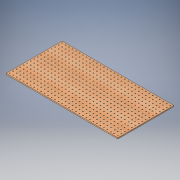
# Autodesk Inventor part: LedBoard
Saved by Autodesk Inventor 2016 (Build 200138000, 138)
## iProperties
Created: 2016-02-08
Part Number: LedBoard
Material: Wood (Birch)
Document SubType Name: Modeling
Designer: ron
Density: 0.55 g/cm^3
Appearance: Birch - Natural Polished
Mass: 4901.48 g
Surface Area: 16574.3 cm^2
Volume: 8911.78 cm^3
Author: ron
Autodesk Inventor part; units mm, degrees
ref_plane "YZ Plane" through (0, 0, 0) normal (1, 0, 0) x (0, 1, 0)
ref_plane "XZ Plane" through (0, 0, 0) normal (0, 1, 0) x (-1, 0, 0)
ref_plane "XY Plane" through (0, 0, 0) normal (0, 0, 1) x (1, 0, 0)
sketch "Sketch1" plane through (0, 0, 0) normal (0, 1, 0) x (-1, 0, 0)
  line L0 (0, 0) -> (1219.2, 0)
  line L1 (1219.2, 0) -> (1219.2, -609.6)
  line L2 (1219.2, -609.6) -> (0, -609.6)
  line L3 (0, -609.6) -> (0, 0)
  circle A0 centre (1200.15, -590.55) radius 5.08
  circle A1 centre (1200.15, -552.45) radius 5.08
  circle A2 centre (1200.15, -514.35) radius 5.08
  circle A3 centre (1200.15, -476.25) radius 5.08
  circle A4 centre (1200.15, -438.15) radius 5.08
  circle A5 centre (1200.15, -400.05) radius 5.08
  circle A6 centre (1200.15, -361.95) radius 5.08
  circle A7 centre (1200.15, -323.85) radius 5.08
  circle A8 centre (1200.15, -285.75) radius 5.08
  circle A9 centre (1200.15, -247.65) radius 5.08
  circle A10 centre (1200.15, -209.55) radius 5.08
  circle A11 centre (1200.15, -171.45) radius 5.08
  circle A12 centre (1200.15, -133.35) radius 5.08
  circle A13 centre (1200.15, -95.25) radius 5.08
  circle A14 centre (1200.15, -57.15) radius 5.08
  circle A15 centre (1200.15, -19.05) radius 5.08
  circle A16 centre (1162.05, -590.55) radius 5.08
  circle A17 centre (1162.05, -552.45) radius 5.08
  circle A18 centre (1162.05, -514.35) radius 5.08
  circle A19 centre (1162.05, -476.25) radius 5.08
  circle A20 centre (1162.05, -438.15) radius 5.08
  circle A21 centre (1162.05, -400.05) radius 5.08
  circle A22 centre (1162.05, -361.95) radius 5.08
  circle A23 centre (1162.05, -323.85) radius 5.08
  circle A24 centre (1162.05, -171.45) radius 5.08
  circle A25 centre (1162.05, -209.55) radius 5.08
  circle A26 centre (1162.05, -247.65) radius 5.08
  circle A27 centre (1162.05, -285.75) radius 5.08
  circle A28 centre (1162.05, -133.35) radius 5.08
  circle A29 centre (1162.05, -95.25) radius 5.08
  circle A30 centre (1162.05, -57.15) radius 5.08
  circle A31 centre (1162.05, -19.05) radius 5.08
  circle A32 centre (1123.95, -590.55) radius 5.08
  circle A33 centre (1123.95, -552.45) radius 5.08
  circle A34 centre (1123.95, -514.35) radius 5.08
  circle A35 centre (1123.95, -476.25) radius 5.08
  circle A36 centre (1123.95, -438.15) radius 5.08
  circle A37 centre (1123.95, -400.05) radius 5.08
  circle A38 centre (1123.95, -361.95) radius 5.08
  circle A39 centre (1123.95, -323.85) radius 5.08
  circle A40 centre (1123.95, -171.45) radius 5.08
  circle A41 centre (1123.95, -209.55) radius 5.08
  circle A42 centre (1123.95, -247.65) radius 5.08
  circle A43 centre (1123.95, -285.75) radius 5.08
  circle A44 centre (1123.95, -133.35) radius 5.08
  circle A45 centre (1123.95, -95.25) radius 5.08
  circle A46 centre (1123.95, -57.15) radius 5.08
  circle A47 centre (1123.95, -19.05) radius 5.08
  circle A48 centre (1085.85, -590.55) radius 5.08
  circle A49 centre (1085.85, -552.45) radius 5.08
  circle A50 centre (1085.85, -514.35) radius 5.08
  circle A51 centre (1085.85, -476.25) radius 5.08
  circle A52 centre (1085.85, -438.15) radius 5.08
  circle A53 centre (1085.85, -400.05) radius 5.08
  circle A54 centre (1085.85, -361.95) radius 5.08
  circle A55 centre (1085.85, -323.85) radius 5.08
  circle A56 centre (1085.85, -171.45) radius 5.08
  circle A57 centre (1085.85, -209.55) radius 5.08
  circle A58 centre (1085.85, -247.65) radius 5.08
  circle A59 centre (1085.85, -285.75) radius 5.08
  circle A60 centre (1085.85, -133.35) radius 5.08
  circle A61 centre (1085.85, -95.25) radius 5.08
  circle A62 centre (1085.85, -57.15) radius 5.08
  circle A63 centre (1085.85, -19.05) radius 5.08
  circle A64 centre (1047.75, -590.55) radius 5.08
  circle A65 centre (1047.75, -552.45) radius 5.08
  circle A66 centre (1047.75, -514.35) radius 5.08
  circle A67 centre (1047.75, -476.25) radius 5.08
  circle A68 centre (1047.75, -438.15) radius 5.08
  circle A69 centre (1047.75, -400.05) radius 5.08
  circle A70 centre (1047.75, -361.95) radius 5.08
  circle A71 centre (1047.75, -323.85) radius 5.08
  circle A72 centre (1047.75, -171.45) radius 5.08
  circle A73 centre (1047.75, -209.55) radius 5.08
  circle A74 centre (1047.75, -247.65) radius 5.08
  circle A75 centre (1047.75, -285.75) radius 5.08
  circle A76 centre (1047.75, -133.35) radius 5.08
  circle A77 centre (1047.75, -95.25) radius 5.08
  circle A78 centre (1047.75, -57.15) radius 5.08
  circle A79 centre (1047.75, -19.05) radius 5.08
  circle A80 centre (1009.65, -590.55) radius 5.08
  circle A81 centre (1009.65, -552.45) radius 5.08
  circle A82 centre (1009.65, -514.35) radius 5.08
  circle A83 centre (1009.65, -476.25) radius 5.08
  circle A84 centre (1009.65, -438.15) radius 5.08
  circle A85 centre (1009.65, -400.05) radius 5.08
  circle A86 centre (1009.65, -361.95) radius 5.08
  circle A87 centre (1009.65, -323.85) radius 5.08
  circle A88 centre (1009.65, -171.45) radius 5.08
  circle A89 centre (1009.65, -209.55) radius 5.08
  circle A90 centre (1009.65, -247.65) radius 5.08
  circle A91 centre (1009.65, -285.75) radius 5.08
  circle A92 centre (1009.65, -133.35) radius 5.08
  circle A93 centre (1009.65, -95.25) radius 5.08
  circle A94 centre (1009.65, -57.15) radius 5.08
  circle A95 centre (1009.65, -19.05) radius 5.08
  circle A96 centre (971.55, -590.55) radius 5.08
  circle A97 centre (971.55, -552.45) radius 5.08
  circle A98 centre (971.55, -514.35) radius 5.08
  circle A99 centre (971.55, -476.25) radius 5.08
  circle A100 centre (971.55, -438.15) radius 5.08
  circle A101 centre (971.55, -400.05) radius 5.08
  circle A102 centre (971.55, -361.95) radius 5.08
  circle A103 centre (971.55, -323.85) radius 5.08
  circle A104 centre (971.55, -171.45) radius 5.08
  circle A105 centre (971.55, -209.55) radius 5.08
  circle A106 centre (971.55, -247.65) radius 5.08
  circle A107 centre (971.55, -285.75) radius 5.08
  circle A108 centre (971.55, -133.35) radius 5.08
  circle A109 centre (971.55, -95.25) radius 5.08
  circle A110 centre (971.55, -57.15) radius 5.08
  circle A111 centre (971.55, -19.05) radius 5.08
  circle A112 centre (933.45, -590.55) radius 5.08
  circle A113 centre (933.45, -552.45) radius 5.08
  circle A114 centre (933.45, -514.35) radius 5.08
  circle A115 centre (933.45, -476.25) radius 5.08
  circle A116 centre (933.45, -438.15) radius 5.08
  circle A117 centre (933.45, -400.05) radius 5.08
  circle A118 centre (933.45, -361.95) radius 5.08
  circle A119 centre (933.45, -323.85) radius 5.08
  circle A120 centre (933.45, -171.45) radius 5.08
  circle A121 centre (933.45, -209.55) radius 5.08
  circle A122 centre (933.45, -247.65) radius 5.08
  circle A123 centre (933.45, -285.75) radius 5.08
  circle A124 centre (933.45, -133.35) radius 5.08
  circle A125 centre (933.45, -95.25) radius 5.08
  circle A126 centre (933.45, -57.15) radius 5.08
  circle A127 centre (933.45, -19.05) radius 5.08
  circle A128 centre (895.35, -590.55) radius 5.08
  circle A129 centre (895.35, -552.45) radius 5.08
  circle A130 centre (895.35, -514.35) radius 5.08
  circle A131 centre (895.35, -476.25) radius 5.08
  circle A132 centre (895.35, -438.15) radius 5.08
  circle A133 centre (895.35, -400.05) radius 5.08
  circle A134 centre (895.35, -361.95) radius 5.08
  circle A135 centre (895.35, -323.85) radius 5.08
  circle A136 centre (895.35, -171.45) radius 5.08
  circle A137 centre (895.35, -209.55) radius 5.08
  circle A138 centre (895.35, -247.65) radius 5.08
  circle A139 centre (895.35, -285.75) radius 5.08
  circle A140 centre (895.35, -133.35) radius 5.08
  circle A141 centre (895.35, -95.25) radius 5.08
  circle A142 centre (895.35, -57.15) radius 5.08
  circle A143 centre (895.35, -19.05) radius 5.08
  circle A144 centre (857.25, -590.55) radius 5.08
  circle A145 centre (857.25, -552.45) radius 5.08
  circle A146 centre (857.25, -514.35) radius 5.08
  circle A147 centre (857.25, -476.25) radius 5.08
  circle A148 centre (857.25, -438.15) radius 5.08
  circle A149 centre (857.25, -400.05) radius 5.08
  circle A150 centre (857.25, -361.95) radius 5.08
  circle A151 centre (857.25, -323.85) radius 5.08
  circle A152 centre (857.25, -171.45) radius 5.08
  circle A153 centre (857.25, -209.55) radius 5.08
  circle A154 centre (857.25, -247.65) radius 5.08
  circle A155 centre (857.25, -285.75) radius 5.08
  circle A156 centre (857.25, -133.35) radius 5.08
  circle A157 centre (857.25, -95.25) radius 5.08
  circle A158 centre (857.25, -57.15) radius 5.08
  circle A159 centre (857.25, -19.05) radius 5.08
  circle A160 centre (819.15, -590.55) radius 5.08
  circle A161 centre (819.15, -552.45) radius 5.08
  circle A162 centre (819.15, -514.35) radius 5.08
  circle A163 centre (819.15, -476.25) radius 5.08
  circle A164 centre (819.15, -438.15) radius 5.08
  circle A165 centre (819.15, -400.05) radius 5.08
  circle A166 centre (819.15, -361.95) radius 5.08
  circle A167 centre (819.15, -323.85) radius 5.08
  circle A168 centre (819.15, -171.45) radius 5.08
  circle A169 centre (819.15, -209.55) radius 5.08
  circle A170 centre (819.15, -247.65) radius 5.08
  circle A171 centre (819.15, -285.75) radius 5.08
  circle A172 centre (819.15, -133.35) radius 5.08
  circle A173 centre (819.15, -95.25) radius 5.08
  circle A174 centre (819.15, -57.15) radius 5.08
  circle A175 centre (819.15, -19.05) radius 5.08
  circle A176 centre (781.05, -590.55) radius 5.08
  circle A177 centre (781.05, -552.45) radius 5.08
  circle A178 centre (781.05, -514.35) radius 5.08
  circle A179 centre (781.05, -476.25) radius 5.08
  circle A180 centre (781.05, -438.15) radius 5.08
  circle A181 centre (781.05, -400.05) radius 5.08
  circle A182 centre (781.05, -361.95) radius 5.08
  circle A183 centre (781.05, -323.85) radius 5.08
  circle A184 centre (781.05, -171.45) radius 5.08
  circle A185 centre (781.05, -209.55) radius 5.08
  circle A186 centre (781.05, -247.65) radius 5.08
  circle A187 centre (781.05, -285.75) radius 5.08
  circle A188 centre (781.05, -133.35) radius 5.08
  circle A189 centre (781.05, -95.25) radius 5.08
  circle A190 centre (781.05, -57.15) radius 5.08
  circle A191 centre (781.05, -19.05) radius 5.08
  circle A192 centre (742.95, -590.55) radius 5.08
  circle A193 centre (742.95, -552.45) radius 5.08
  circle A194 centre (742.95, -514.35) radius 5.08
  circle A195 centre (742.95, -476.25) radius 5.08
  circle A196 centre (742.95, -438.15) radius 5.08
  circle A197 centre (742.95, -400.05) radius 5.08
  circle A198 centre (742.95, -361.95) radius 5.08
  circle A199 centre (742.95, -323.85) radius 5.08
  circle A200 centre (742.95, -171.45) radius 5.08
  circle A201 centre (742.95, -209.55) radius 5.08
  circle A202 centre (742.95, -247.65) radius 5.08
  circle A203 centre (742.95, -285.75) radius 5.08
  circle A204 centre (742.95, -133.35) radius 5.08
  circle A205 centre (742.95, -95.25) radius 5.08
  circle A206 centre (742.95, -57.15) radius 5.08
  circle A207 centre (742.95, -19.05) radius 5.08
  circle A208 centre (704.85, -590.55) radius 5.08
  circle A209 centre (704.85, -552.45) radius 5.08
  circle A210 centre (704.85, -514.35) radius 5.08
  circle A211 centre (704.85, -476.25) radius 5.08
  circle A212 centre (704.85, -438.15) radius 5.08
  circle A213 centre (704.85, -400.05) radius 5.08
  circle A214 centre (704.85, -361.95) radius 5.08
  circle A215 centre (704.85, -323.85) radius 5.08
  circle A216 centre (704.85, -171.45) radius 5.08
  circle A217 centre (704.85, -209.55) radius 5.08
  circle A218 centre (704.85, -247.65) radius 5.08
  circle A219 centre (704.85, -285.75) radius 5.08
  circle A220 centre (704.85, -133.35) radius 5.08
  circle A221 centre (704.85, -95.25) radius 5.08
  circle A222 centre (704.85, -57.15) radius 5.08
  circle A223 centre (704.85, -19.05) radius 5.08
  circle A224 centre (666.75, -590.55) radius 5.08
  circle A225 centre (666.75, -552.45) radius 5.08
  circle A226 centre (666.75, -514.35) radius 5.08
  circle A227 centre (666.75, -476.25) radius 5.08
  circle A228 centre (666.75, -438.15) radius 5.08
  circle A229 centre (666.75, -400.05) radius 5.08
  circle A230 centre (666.75, -361.95) radius 5.08
  circle A231 centre (666.75, -323.85) radius 5.08
  circle A232 centre (666.75, -171.45) radius 5.08
  circle A233 centre (666.75, -209.55) radius 5.08
  circle A234 centre (666.75, -247.65) radius 5.08
  circle A235 centre (666.75, -285.75) radius 5.08
  circle A236 centre (666.75, -133.35) radius 5.08
  circle A237 centre (666.75, -95.25) radius 5.08
  circle A238 centre (666.75, -57.15) radius 5.08
  circle A239 centre (666.75, -19.05) radius 5.08
  circle A240 centre (19.05, -590.55) radius 5.08
  circle A241 centre (19.05, -552.45) radius 5.08
  circle A242 centre (19.05, -514.35) radius 5.08
  circle A243 centre (19.05, -476.25) radius 5.08
  circle A244 centre (19.05, -438.15) radius 5.08
  circle A245 centre (19.05, -400.05) radius 5.08
  circle A246 centre (19.05, -361.95) radius 5.08
  circle A247 centre (19.05, -323.85) radius 5.08
  circle A248 centre (19.05, -171.45) radius 5.08
  circle A249 centre (19.05, -209.55) radius 5.08
  circle A250 centre (19.05, -247.65) radius 5.08
  circle A251 centre (19.05, -285.75) radius 5.08
  circle A252 centre (19.05, -133.35) radius 5.08
  circle A253 centre (19.05, -95.25) radius 5.08
  circle A254 centre (19.05, -57.15) radius 5.08
  circle A255 centre (19.05, -19.05) radius 5.08
  circle A256 centre (57.15, -590.55) radius 5.08
  circle A257 centre (60.8018, -552.45) radius 5.08
  circle A258 centre (60.8018, -514.35) radius 5.08
  circle A259 centre (60.8018, -476.25) radius 5.08
  circle A260 centre (60.8018, -438.15) radius 5.08
  circle A261 centre (60.8018, -400.05) radius 5.08
  circle A262 centre (60.8018, -361.95) radius 5.08
  circle A263 centre (60.8018, -323.85) radius 5.08
  circle A264 centre (60.8018, -171.45) radius 5.08
  circle A265 centre (60.8018, -209.55) radius 5.08
  circle A266 centre (60.8018, -247.65) radius 5.08
  circle A267 centre (60.8018, -285.75) radius 5.08
  circle A268 centre (60.8018, -133.35) radius 5.08
  circle A269 centre (60.8018, -95.25) radius 5.08
  circle A270 centre (60.8018, -57.15) radius 5.08
  circle A271 centre (60.8018, -19.05) radius 5.08
  circle A272 centre (590.55, -590.55) radius 5.08
  circle A273 centre (590.55, -552.45) radius 5.08
  circle A274 centre (590.55, -514.35) radius 5.08
  circle A275 centre (590.55, -476.25) radius 5.08
  circle A276 centre (590.55, -438.15) radius 5.08
  circle A277 centre (590.55, -400.05) radius 5.08
  circle A278 centre (590.55, -361.95) radius 5.08
  circle A279 centre (590.55, -323.85) radius 5.08
  circle A280 centre (590.55, -171.45) radius 5.08
  circle A281 centre (590.55, -209.55) radius 5.08
  circle A282 centre (590.55, -247.65) radius 5.08
  circle A283 centre (590.55, -285.75) radius 5.08
  circle A284 centre (590.55, -133.35) radius 5.08
  circle A285 centre (590.55, -95.25) radius 5.08
  circle A286 centre (590.55, -57.15) radius 5.08
  circle A287 centre (590.55, -19.05) radius 5.08
  circle A288 centre (552.45, -590.55) radius 5.08
  circle A289 centre (552.45, -552.45) radius 5.08
  circle A290 centre (552.45, -514.35) radius 5.08
  circle A291 centre (552.45, -476.25) radius 5.08
  circle A292 centre (552.45, -438.15) radius 5.08
  circle A293 centre (552.45, -400.05) radius 5.08
  circle A294 centre (552.45, -361.95) radius 5.08
  circle A295 centre (552.45, -323.85) radius 5.08
  circle A296 centre (552.45, -171.45) radius 5.08
  circle A297 centre (552.45, -209.55) radius 5.08
  circle A298 centre (552.45, -247.65) radius 5.08
  circle A299 centre (552.45, -285.75) radius 5.08
  circle A300 centre (552.45, -133.35) radius 5.08
  circle A301 centre (552.45, -95.25) radius 5.08
  circle A302 centre (552.45, -57.15) radius 5.08
  circle A303 centre (552.45, -19.05) radius 5.08
  circle A304 centre (95.25, -590.55) radius 5.08
  circle A305 centre (92.3807, -552.45) radius 5.08
  circle A306 centre (92.3807, -514.35) radius 5.08
  circle A307 centre (92.3807, -476.25) radius 5.08
  circle A308 centre (92.3807, -438.15) radius 5.08
  circle A309 centre (92.3807, -400.05) radius 5.08
  circle A310 centre (92.3807, -361.95) radius 5.08
  circle A311 centre (92.3807, -323.85) radius 5.08
  circle A312 centre (92.3807, -171.45) radius 5.08
  circle A313 centre (92.3807, -209.55) radius 5.08
  circle A314 centre (92.3807, -247.65) radius 5.08
  circle A315 centre (92.3807, -285.75) radius 5.08
  circle A316 centre (92.3807, -133.35) radius 5.08
  circle A317 centre (92.3807, -95.25) radius 5.08
  circle A318 centre (92.3807, -57.15) radius 5.08
  circle A319 centre (92.3807, -19.05) radius 5.08
  circle A320 centre (514.35, -590.55) radius 5.08
  circle A321 centre (514.35, -552.45) radius 5.08
  circle A322 centre (514.35, -514.35) radius 5.08
  circle A323 centre (514.35, -476.25) radius 5.08
  circle A324 centre (514.35, -438.15) radius 5.08
  circle A325 centre (514.35, -400.05) radius 5.08
  circle A326 centre (514.35, -361.95) radius 5.08
  circle A327 centre (514.35, -323.85) radius 5.08
  circle A328 centre (514.35, -171.45) radius 5.08
  circle A329 centre (514.35, -209.55) radius 5.08
  circle A330 centre (514.35, -247.65) radius 5.08
  circle A331 centre (514.35, -285.75) radius 5.08
  circle A332 centre (514.35, -133.35) radius 5.08
  circle A333 centre (514.35, -95.25) radius 5.08
  circle A334 centre (514.35, -57.15) radius 5.08
  circle A335 centre (514.35, -19.05) radius 5.08
  circle A336 centre (133.35, -590.55) radius 5.08
  circle A337 centre (133.35, -552.45) radius 5.08
  circle A338 centre (133.35, -514.35) radius 5.08
  circle A339 centre (133.35, -476.25) radius 5.08
  circle A340 centre (133.35, -438.15) radius 5.08
  circle A341 centre (133.35, -400.05) radius 5.08
  circle A342 centre (133.35, -361.95) radius 5.08
  circle A343 centre (133.35, -323.85) radius 5.08
  circle A344 centre (133.35, -171.45) radius 5.08
  circle A345 centre (133.35, -209.55) radius 5.08
  circle A346 centre (133.35, -247.65) radius 5.08
  circle A347 centre (133.35, -285.75) radius 5.08
  circle A348 centre (133.35, -133.35) radius 5.08
  circle A349 centre (133.35, -95.25) radius 5.08
  circle A350 centre (133.35, -57.15) radius 5.08
  circle A351 centre (133.35, -19.05) radius 5.08
  circle A352 centre (476.25, -590.55) radius 5.08
  circle A353 centre (476.25, -552.45) radius 5.08
  circle A354 centre (476.25, -514.35) radius 5.08
  circle A355 centre (476.25, -476.25) radius 5.08
  circle A356 centre (476.25, -438.15) radius 5.08
  circle A357 centre (476.25, -400.05) radius 5.08
  circle A358 centre (476.25, -361.95) radius 5.08
  circle A359 centre (476.25, -323.85) radius 5.08
  circle A360 centre (476.25, -171.45) radius 5.08
  circle A361 centre (476.25, -209.55) radius 5.08
  circle A362 centre (476.25, -247.65) radius 5.08
  circle A363 centre (476.25, -285.75) radius 5.08
  circle A364 centre (476.25, -133.35) radius 5.08
  circle A365 centre (476.25, -95.25) radius 5.08
  circle A366 centre (476.25, -57.15) radius 5.08
  circle A367 centre (476.25, -19.05) radius 5.08
  circle A368 centre (438.15, -590.55) radius 5.08
  circle A369 centre (438.15, -552.45) radius 5.08
  circle A370 centre (438.15, -514.35) radius 5.08
  circle A371 centre (438.15, -476.25) radius 5.08
  circle A372 centre (438.15, -438.15) radius 5.08
  circle A373 centre (438.15, -400.05) radius 5.08
  circle A374 centre (438.15, -361.95) radius 5.08
  circle A375 centre (438.15, -323.85) radius 5.08
  circle A376 centre (438.15, -171.45) radius 5.08
  circle A377 centre (438.15, -209.55) radius 5.08
  circle A378 centre (438.15, -247.65) radius 5.08
  circle A379 centre (438.15, -285.75) radius 5.08
  circle A380 centre (438.15, -133.35) radius 5.08
  circle A381 centre (438.15, -95.25) radius 5.08
  circle A382 centre (438.15, -57.15) radius 5.08
  circle A383 centre (438.15, -19.05) radius 5.08
  circle A384 centre (400.05, -590.55) radius 5.08
  circle A385 centre (400.05, -552.45) radius 5.08
  circle A386 centre (400.05, -514.35) radius 5.08
  circle A387 centre (400.05, -476.25) radius 5.08
  circle A388 centre (400.05, -438.15) radius 5.08
  circle A389 centre (400.05, -400.05) radius 5.08
  circle A390 centre (400.05, -361.95) radius 5.08
  circle A391 centre (400.05, -323.85) radius 5.08
  circle A392 centre (400.05, -171.45) radius 5.08
  circle A393 centre (400.05, -209.55) radius 5.08
  circle A394 centre (400.05, -247.65) radius 5.08
  circle A395 centre (400.05, -285.75) radius 5.08
  circle A396 centre (400.05, -133.35) radius 5.08
  circle A397 centre (400.05, -95.25) radius 5.08
  circle A398 centre (400.05, -57.15) radius 5.08
  circle A399 centre (400.05, -19.05) radius 5.08
  circle A400 centre (171.45, -590.55) radius 5.08
  circle A401 centre (171.45, -552.45) radius 5.08
  circle A402 centre (171.45, -514.35) radius 5.08
  circle A403 centre (171.45, -476.25) radius 5.08
  circle A404 centre (171.45, -438.15) radius 5.08
  circle A405 centre (171.45, -400.05) radius 5.08
  circle A406 centre (171.45, -361.95) radius 5.08
  circle A407 centre (171.45, -323.85) radius 5.08
  circle A408 centre (171.45, -171.45) radius 5.08
  circle A409 centre (171.45, -209.55) radius 5.08
  circle A410 centre (171.45, -247.65) radius 5.08
  circle A411 centre (171.45, -285.75) radius 5.08
  circle A412 centre (171.45, -133.35) radius 5.08
  circle A413 centre (171.45, -95.25) radius 5.08
  circle A414 centre (171.45, -57.15) radius 5.08
  circle A415 centre (171.45, -19.05) radius 5.08
  circle A416 centre (361.95, -590.55) radius 5.08
  circle A417 centre (361.95, -552.45) radius 5.08
  circle A418 centre (361.95, -514.35) radius 5.08
  circle A419 centre (361.95, -476.25) radius 5.08
  circle A420 centre (361.95, -438.15) radius 5.08
  circle A421 centre (361.95, -400.05) radius 5.08
  circle A422 centre (361.95, -361.95) radius 5.08
  circle A423 centre (361.95, -323.85) radius 5.08
  circle A424 centre (361.95, -171.45) radius 5.08
  circle A425 centre (361.95, -209.55) radius 5.08
  circle A426 centre (361.95, -247.65) radius 5.08
  circle A427 centre (361.95, -285.75) radius 5.08
  circle A428 centre (361.95, -133.35) radius 5.08
  circle A429 centre (361.95, -95.25) radius 5.08
  circle A430 centre (361.95, -57.15) radius 5.08
  circle A431 centre (361.95, -19.05) radius 5.08
  circle A432 centre (323.85, -590.55) radius 5.08
  circle A433 centre (323.85, -552.45) radius 5.08
  circle A434 centre (323.85, -514.35) radius 5.08
  circle A435 centre (323.85, -476.25) radius 5.08
  circle A436 centre (323.85, -438.15) radius 5.08
  circle A437 centre (323.85, -400.05) radius 5.08
  circle A438 centre (323.85, -361.95) radius 5.08
  circle A439 centre (323.85, -323.85) radius 5.08
  circle A440 centre (323.85, -171.45) radius 5.08
  circle A441 centre (323.85, -209.55) radius 5.08
  circle A442 centre (323.85, -247.65) radius 5.08
  circle A443 centre (323.85, -285.75) radius 5.08
  circle A444 centre (323.85, -133.35) radius 5.08
  circle A445 centre (323.85, -95.25) radius 5.08
  circle A446 centre (323.85, -57.15) radius 5.08
  circle A447 centre (323.85, -19.05) radius 5.08
  circle A448 centre (209.55, -590.55) radius 5.08
  circle A449 centre (206.3715, -552.45) radius 5.08
  circle A450 centre (211.3282, -514.6738) radius 5.08
  circle A451 centre (211.3282, -476.5738) radius 5.08
  circle A452 centre (211.3282, -438.4738) radius 5.08
  circle A453 centre (211.3282, -400.3738) radius 5.08
  circle A454 centre (211.3282, -362.2738) radius 5.08
  circle A455 centre (211.3282, -324.1738) radius 5.08
  circle A456 centre (211.3282, -171.7738) radius 5.08
  circle A457 centre (211.3282, -209.8738) radius 5.08
  circle A458 centre (211.3282, -247.9738) radius 5.08
  circle A459 centre (211.3282, -286.0738) radius 5.08
  circle A460 centre (211.3282, -133.6738) radius 5.08
  circle A461 centre (211.3282, -95.5738) radius 5.08
  circle A462 centre (211.3282, -57.4738) radius 5.08
  circle A463 centre (211.3282, -19.3738) radius 5.08
  circle A464 centre (285.75, -590.55) radius 5.08
  circle A465 centre (285.75, -552.45) radius 5.08
  circle A466 centre (285.75, -514.35) radius 5.08
  circle A467 centre (285.75, -476.25) radius 5.08
  circle A468 centre (285.75, -438.15) radius 5.08
  circle A469 centre (285.75, -400.05) radius 5.08
  circle A470 centre (285.75, -361.95) radius 5.08
  circle A471 centre (285.75, -323.85) radius 5.08
  circle A472 centre (285.75, -171.45) radius 5.08
  circle A473 centre (285.75, -209.55) radius 5.08
  circle A474 centre (285.75, -247.65) radius 5.08
  circle A475 centre (285.75, -285.75) radius 5.08
  circle A476 centre (285.75, -133.35) radius 5.08
  circle A477 centre (285.75, -95.25) radius 5.08
  circle A478 centre (285.75, -57.15) radius 5.08
  circle A479 centre (285.75, -19.05) radius 5.08
  circle A480 centre (247.65, -590.55) radius 5.08
  circle A481 centre (247.65, -552.45) radius 5.08
  circle A482 centre (247.65, -514.35) radius 5.08
  circle A483 centre (247.65, -476.25) radius 5.08
  circle A484 centre (247.65, -438.15) radius 5.08
  circle A485 centre (247.65, -400.05) radius 5.08
  circle A486 centre (247.65, -361.95) radius 5.08
  circle A487 centre (247.65, -323.85) radius 5.08
  circle A488 centre (247.65, -171.45) radius 5.08
  circle A489 centre (247.65, -209.55) radius 5.08
  circle A490 centre (247.65, -247.65) radius 5.08
  circle A491 centre (247.65, -285.75) radius 5.08
  circle A492 centre (247.65, -133.35) radius 5.08
  circle A493 centre (247.65, -95.25) radius 5.08
  circle A494 centre (247.65, -57.15) radius 5.08
  circle A495 centre (247.65, -19.05) radius 5.08
  circle A496 centre (628.65, -95.25) radius 5.08
  circle A497 centre (628.65, -19.05) radius 5.08
  circle A498 centre (628.65, -133.35) radius 5.08
  circle A499 centre (628.65, -171.45) radius 5.08
  circle A500 centre (628.65, -209.55) radius 5.08
  circle A501 centre (628.65, -247.65) radius 5.08
  circle A502 centre (628.65, -285.75) radius 5.08
  circle A503 centre (628.65, -323.85) radius 5.08
  circle A504 centre (628.65, -361.95) radius 5.08
  circle A505 centre (628.65, -400.05) radius 5.08
  circle A506 centre (628.65, -438.15) radius 5.08
  circle A507 centre (628.65, -476.25) radius 5.08
  circle A508 centre (628.65, -552.45) radius 5.08
  circle A509 centre (628.65, -590.55) radius 5.08
  circle A510 centre (628.65, -514.35) radius 5.08
  circle A511 centre (628.65, -57.15) radius 5.08
  dimension "d0" = 1219.2
  dimension "d1" = 609.6
  dimension "d4" = 10.16
  dimension "d5" = 19.05
  dimension "d6" = 19.05
  dimension "d7" = 10.16
  dimension "d8" = 38.1
  dimension "d9" = 19.05
  dimension "d10" = 10.16
  dimension "d11" = 10.16
  dimension "d12" = 38.1
  dimension "d13" = 10.16
  dimension "d14" = 10.16
  dimension "d15" = 38.1
  dimension "d16" = 10.16
  dimension "d17" = 10.16
  dimension "d18" = 38.1
  dimension "d19" = 38.1
  dimension "d20" = 38.1
  dimension "d21" = 38.1
  dimension "d22" = 10.16
  dimension "d23" = 10.16
  dimension "d24" = 38.1
  dimension "d25" = 10.16
  dimension "d26" = 10.16
  dimension "d27" = 38.1
  dimension "d28" = 10.16
  dimension "d29" = 10.16
  dimension "d30" = 38.1
  dimension "d31" = 10.16
  dimension "d32" = 10.16
  dimension "d33" = 38.1
  dimension "d34" = 38.1
  dimension "d35" = 38.1
  dimension "d36" = 38.1
  dimension "d37" = 38.1
  dimension "d38" = 19.05
  dimension "d39" = 19.05
  dimension "d40" = 19.05
  dimension "d41" = 19.05
  dimension "d42" = 19.05
  dimension "d43" = 19.05
  dimension "d44" = 19.05
  dimension "d45" = 19.05
  dimension "d46" = 19.05
  dimension "d47" = 19.05
  dimension "d48" = 19.05
  dimension "d49" = 19.05
  dimension "d50" = 19.05
  dimension "d51" = 19.05
  dimension "d52" = 10.16
  dimension "d53" = 10.16
  dimension "d54" = 38.1
  dimension "d55" = 10.16
  dimension "d56" = 10.16
  dimension "d57" = 38.1
  dimension "d58" = 10.16
  dimension "d59" = 10.16
  dimension "d60" = 38.1
  dimension "d61" = 10.16
  dimension "d62" = 10.16
  dimension "d63" = 38.1
  dimension "d64" = 38.1
  dimension "d65" = 38.1
  constraints: 512 centre point, 8 end point, 2 parallel, 1 horizontal, 1 perpendicular
  measures "d0" distance of L1.end L2.end
  measures "d1" distance of L2.end L0.start
  measures "d4" diameter of A0
  measures "d5" distance from line of L2 A0.centre
  measures "d6" distance from line of L1 A0.centre
  measures "d7" diameter of A1
  measures "d8" distance of A0.centre A1.centre
  measures "d9" distance from line of L1 A1.centre
  measures "d10" diameter of A2
  measures "d11" diameter of A3
  measures "d12" distance of A2.centre A3.centre
  measures "d13" diameter of A4
  measures "d14" diameter of A5
  measures "d15" distance of A4.centre A5.centre
  measures "d16" diameter of A6
  measures "d17" diameter of A7
  measures "d18" distance of A6.centre A7.centre
  measures "d19" distance of A1.centre A2.centre
  measures "d20" distance of A3.centre A4.centre
  measures "d21" distance of A5.centre A6.centre
  measures "d22" diameter of A8
  measures "d23" diameter of A9
  measures "d24" distance of A8.centre A9.centre
  measures "d25" diameter of A10
  measures "d26" diameter of A11
  measures "d27" distance of A10.centre A11.centre
  measures "d28" diameter of A12
  measures "d29" diameter of A13
  measures "d30" distance of A12.centre A13.centre
  measures "d31" diameter of A14
  measures "d32" diameter of A15
  measures "d33" distance of A14.centre A15.centre
  measures "d34" distance of A9.centre A10.centre
  measures "d35" distance of A11.centre A12.centre
  measures "d36" distance of A13.centre A14.centre
  measures "d37" distance of A7.centre A8.centre
  measures "d38" distance from line of L1 A15.centre
  measures "d39" distance from line of A15.centre L0
  measures "d40" distance from line of A14.centre L1
  measures "d41" distance from line of A13.centre L1
  measures "d42" distance from line of A12.centre L1
  measures "d43" distance from line of A11.centre L1
  measures "d44" distance from line of A10.centre L1
  measures "d45" distance from line of A9.centre L1
  measures "d46" distance from line of A8.centre L1
  measures "d47" distance from line of A7.centre L1
  measures "d48" distance from line of A6.centre L1
  measures "d49" distance from line of A5.centre L1
  measures "d50" distance from line of A4.centre L1
  measures "d51" distance from line of A3.centre L1
  measures "d52" diameter of A16
  measures "d53" diameter of A17
  measures "d54" distance of A16.centre A17.centre
  measures "d55" diameter of A18
  measures "d56" diameter of A19
  measures "d57" distance of A18.centre A19.centre
  measures "d58" diameter of A20
  measures "d59" diameter of A21
  measures "d60" distance of A20.centre A21.centre
  measures "d61" diameter of A22
  measures "d62" diameter of A23
  measures "d63" distance of A22.centre A23.centre
  measures "d64" distance of A17.centre A18.centre
  measures "d65" distance of A19.centre A20.centre
extrude "Extrusion3" add sketch "Sketch1" along normal blind 12.7
body "Solid3"
